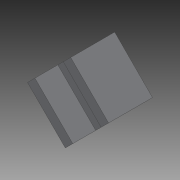
# Autodesk Inventor part: eye_cam_arm_brace
Saved by Autodesk Inventor 2015 (Build 190159000, 159)
## iProperties
Created: 2015-06-21
Part Number: eye_cam_arm_brace
Material: Generic
Document SubType Name: Modeling
Designer: Master
Density: 1 g/cm^3
Appearance: Default
Author: Master
Autodesk Inventor part; units mm, degrees
ref_plane "YZ Plane" through (0, 0, 0) normal (1, 0, 0) x (0, 1, 0)
ref_plane "XZ Plane" through (0, 0, 0) normal (0, 1, 0) x (-1, 0, 0)
ref_plane "XY Plane" through (0, 0, 0) normal (0, 0, 1) x (1, 0, 0)
sketch "Sketch1" plane through (0, 0, 0) normal (0, 0, 1) x (1, 0, 0)
  circle A0 centre (43.3303, -43.3303) radius 1.5 projected
  circle A1 centre (32.0698, -32.0698) radius 1.5 projected
  arc A2 (2.3181, 4.753) -> (-4.753, -2.3181) centre (-1.2174, 1.2174) ccw projected
  line L0 (-4.753, -2.3181) -> (44.7445, -51.8156) projected
  line L1 (44.7445, -51.8156) -> (51.8156, -44.7445) projected
  line L2 (51.8156, -44.7445) -> (2.3181, 4.753) projected
  line L3 (44.7445, -51.8156) -> (34.845, -41.9161)
  line L4 (44.7445, -51.8156) -> (51.8156, -44.7445)
  line L5 (51.8156, -44.7445) -> (41.9161, -34.845)
  line L6 (34.845, -41.9161) -> (41.9161, -34.845)
  line L7 (44.7445, -51.8156) -> (42.6232, -53.9369)
  line L8 (42.6232, -53.9369) -> (32.7237, -44.0374)
  line L9 (32.7237, -44.0374) -> (34.845, -41.9161)
  line L10 (51.8156, -44.7445) -> (53.9369, -42.6232)
  line L11 (53.9369, -42.6232) -> (44.0374, -32.7237)
  line L12 (44.0374, -32.7237) -> (41.9161, -34.845)
  line L13 (44.391, -52.1691) -> (34.4915, -42.2697)
  line L14 (52.1691, -44.391) -> (42.2697, -34.4915)
  point P0 (0, 0)
  dimension "d1" = 7
  dimension "d2" = 3
  dimension "d3" = 3
  dimension "d10" = 0.5
  dimension "d11" = 0.5
  constraints: 24 end point, 8 point on line, 2 parallel
  measures "d1" distance from line of L6 A0.centre
  measures "d2" distance between parallel lines of L0 L8
  measures "d3" distance between parallel lines of L2 L11
  measures "d10" distance between parallel lines of L13 L0
  measures "d11" distance between parallel lines of L2 L14
extrude "Extrusion1" add sketch "Sketch1" along normal blind 2.5 contours L12 L14 L10 L2 | L2 L1 L0 L6 | L0 L7 L13 L9 | L12 L11 L10 L14 | L13 L7 L8 L9
sketch "Sketch2" plane through (0, 0, 0) normal (0, 0, -1) x (-1, 0, 0)
  line L0 (-32.7237, -44.0374) -> (-42.6232, -53.9369) projected
  line L1 (4.753, -2.3181) -> (-44.7445, -51.8156) projected
  line L2 (-42.6232, -53.9369) -> (-44.7445, -51.8156) projected
  line L3 (-44.0374, -32.7237) -> (-32.7237, -44.0374) projected
  line L4 (-53.9369, -42.6232) -> (-44.0374, -32.7237) projected
  line L5 (-51.8156, -44.7445) -> (-2.3181, 4.753) projected
  line L6 (-51.8156, -44.7445) -> (-53.9369, -42.6232) projected
  line L7 (-32.7237, -44.0374) -> (-34.845, -41.9161)
  line L8 (-44.0374, -32.7237) -> (-32.7237, -44.0374) projected
  line L9 (-44.0374, -32.7237) -> (-41.9161, -34.845)
  line L10 (-34.6683, -42.0929) -> (-44.5677, -51.9924)
  line L11 (-42.0929, -34.6683) -> (-51.9924, -44.5677)
  point P0 (0, 0)
  dimension "d12" = 0.25
  dimension "d13" = 0.25
  constraints: 8 end point, 8 point on line
  measures "d12" distance between parallel lines of L10 L1
  measures "d13" distance between parallel lines of L5 L11
extrude "Extrusion2" add sketch "Sketch2" along normal blind 3 contours L0 L2 L10 L3 | L11 L6 L4 L3
sketch "Sketch3" plane through (0, 0, 2.5) normal (0, 0, 1) x (1, 0, 0)
  line L0 (-4.753, -2.3181) -> (44.7445, -51.8156) projected
  line L1 (42.6232, -53.9369) -> (44.7445, -51.8156) projected
  line L2 (32.7237, -44.0374) -> (42.6232, -53.9369) projected
  line L3 (53.9369, -42.6232) -> (44.0374, -32.7237) projected
  line L4 (51.8156, -44.7445) -> (53.9369, -42.6232) projected
  line L5 (51.8156, -44.7445) -> (2.3181, 4.753) projected
  line L6 (41.9161, -34.845) -> (44.0374, -32.7237)
  line L7 (51.9924, -44.5677) -> (42.0929, -34.6683) projected
  line L8 (34.6683, -42.0929) -> (44.5677, -51.9924) projected
  line L9 (34.6683, -42.0929) -> (32.7237, -44.0374)
  line L10 (44.0374, -32.7237) -> (32.7237, -44.0374) projected
  point P0 (0, 0)
  constraints: 4 end point, 3 point on line
extrude "Extrusion3" add sketch "Sketch3" along normal blind 6 contours L8 L1 L2 L9 | L6 L3 L4 L7
body "Solid1"
